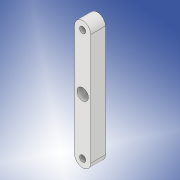
# Autodesk Inventor part: WaveGenerator
Saved by Autodesk Inventor 2017 (Build 210142000, 142)
## iProperties
Created: 2017-07-11
Part Number: WaveGenerator
Material: ABS Plastic
Document SubType Name: Modeling
Designer: zallen
Density: 1.06 g/cm^3
Appearance: CR White
Author: zallen
Autodesk Inventor part; units mm, degrees
ref_plane "YZ Plane" through (0, 0, 0) normal (1, 0, 0) x (0, 1, 0)
ref_plane "XZ Plane" through (0, 0, 0) normal (0, 1, 0) x (-1, 0, 0)
ref_plane "XY Plane" through (0, 0, 0) normal (0, 0, 1) x (1, 0, 0)
sketch "Sketch1" plane through (0, 0, 0) normal (0, 0, 1) x (1, 0, 0)
  line L0 (0, 0) -> (0, 87) construction
  circle A0 centre (0, 81.5) radius 5.5 construction
  circle A1 centre (0, 5.5) radius 5.5 construction
  line L1 (5.5, 81.5) -> (5.5, 5.5)
  line L2 (-5.5, 5.5) -> (-5.5, 81.5)
  arc A2 (5.5, 81.5) -> (-5.5, 81.5) centre (0, 81.5) ccw
  arc A3 (-5.5, 5.5) -> (5.5, 5.5) centre (0, 5.5) ccw
  circle A4 centre (0, 43.5) radius 3.9
  circle A5 centre (0, 81.5) radius 2.1
  circle A6 centre (0, 5.5) radius 2.1
  dimension "d0" = 87
  dimension "d1" = 11
  dimension "d2" = 11
  dimension "d3" = 7.8
  dimension "d4" = 4.2
  dimension "d5" = 4.2
  constraints: 10 point on circle, 7 centre point, 6 end point, 6 tangent, 2 coincident, 2 point on line, 1 concentric, 1 midpoint, 1 vertical
  measures "d0" distance of L0.start L0.end
  measures "d1" diameter of A0
  measures "d2" diameter of A1
  measures "d3" diameter of A4
  measures "d4" diameter of A5
  measures "d5" diameter of A6
extrude "Extrusion1" add sketch "Sketch1" along normal blind 10
body "Solid1"
